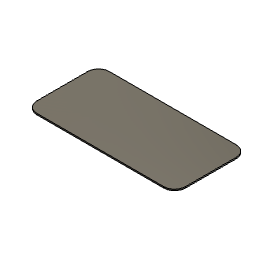
Component12 (Autodesk Fusion 360 design; units mm, degrees)
Autodesk Fusion 360 part; units mm, degrees
sketch "Sketch1" plane through (0, -40, 0) normal (0, -1, 0) x (1, 0, 0)
  line L0 (138.45, 65) -> (138.45, -65)
  line L1 (138.45, -65) -> (141.95, -65)
  line L2 (141.95, -65) -> (141.95, 65)
  line L3 (141.95, 65) -> (138.45, 65)
  line L4 (12.2662, -100) -> (362.2662, -100)
  line L5 (392.2662, -70) -> (392.2662, 70)
  line L6 (362.2662, 100) -> (12.2662, 100)
  line L7 (-17.7338, 70) -> (-17.7338, -70)
  line L8 (-17.7338, -100) -> (392.2662, 100) construction
  line L9 (392.2662, -100) -> (-17.7338, 100) construction
  arc A0 (12.2662, 100) -> (-17.7338, 70) centre (12.2662, 70) ccw
  arc A1 (-17.7338, -70) -> (12.2662, -100) centre (12.2662, -70) ccw
  arc A2 (362.2662, -100) -> (392.2662, -70) centre (362.2662, -70) ccw
  arc A3 (392.2662, 70) -> (362.2662, 100) centre (362.2662, 70) ccw
  point P0 (187.2662, 0)
  dimension "d153" = 410
  dimension "d154" = 30
  constraint horizontal L4
  constraint perpendicular L4 L5
  constraint parallel L4 L6
  constraint parallel L5 L7
  constraint coincident L8 P0
  constraint coincident L9 P0
  constraint coincident L9.end L6
  constraint coincident L9.end L7
  constraint tangent L6 A0
  constraint tangent L7 A0
  constraint coincident L8.start L7
  constraint coincident L8.start L4
  constraint tangent L7 A1
  constraint tangent L4 A1
  constraint equal A0 A1
  constraint coincident L9.start L4
  constraint coincident L9.start L5
  constraint tangent L4 A2
  constraint tangent L5 A2
  constraint equal A0 A2
  constraint coincident L8.end L6
  constraint coincident L8.end L5
  constraint tangent L6 A3
  constraint tangent L5 A3
  constraint equal A0 A3
  measures "d153" distance of L8.end L9.end
  measures "d154" radius of A0
extrude "Extrude1" add sketch "Sketch1" along normal blind 3.5 contours L0 L1 L2 L3 | L4 L5 L6 L7 A0 A1 A2 A3
